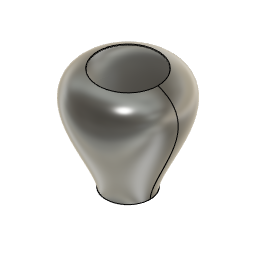
Vase_Homework (Autodesk Fusion 360 design; units mm, degrees)
Autodesk Fusion 360 part; units mm, degrees
sketch "Vase_Form" plane through (0, 0, 0) normal (0, 1, 0) x (1, 0, 0)
  spline S0 degree 5 poles (51.5187, 0) (51.5848, -1.6112) (51.9328, -5.0874) (53.1023, -11.0626) (55.9659, -20.5625) (61.704, -35.0058) (69.4537, -51.9393) (78.8368, -71.1094) (89.1317, -91.9905) (99.3864, -113.8767) (108.5272, -135.9665) (115.4599, -157.4412) (119.1828, -177.5466) (118.8878, -195.6666) (114.1203, -211.4335) (104.7239, -224.693) (93.5064, -233.2688) (83.0443, -238.5707) (75.1654, -241.6067) (71, -243) knots 0 0 0 0 0 0 0.066667 0.133333 0.2 0.266667 0.333333 0.4 0.466667 0.533333 0.6 0.666667 0.733333 0.8 0.866667 0.933333 1 1 1 1 1 1
  spline S1 degree 3 poles (53.0174, 0.0615) (53.2384, -5.3236) (55.0217, -12.7462) (58.4146, -22.0874) (61.2187, -29.8075) (65.129, -38.8618) (69.9141, -49.0892) (74.7583, -59.4428) (80.504, -71.0046) (86.4594, -83.2675) (94.4824, -99.7881) (102.8561, -117.5556) (109.2126, -134.8292) (114.0806, -148.0578) (117.7392, -160.9765) (119.248, -172.9258) (120.6759, -184.2343) (120.1641, -194.6786) (117.2946, -203.9293) (114.1604, -214.0334) (108.219, -222.6945) (99.5527, -229.7433) (92.1398, -235.7726) (82.7612, -240.6476) (71.4758, -244.4225) knots 0 0 0 0 0.140334 0.140334 0.140334 0.256315 0.256315 0.256315 0.373727 0.373727 0.373727 0.531903 0.531903 0.531903 0.653038 0.653038 0.653038 0.767678 0.767678 0.767678 0.892894 0.892894 0.892894 1 1 1 1
  spline S2 degree 5 poles (71, -243) (70.9155, -243.0511) (70.7546, -243.1512) (70.5382, -243.2955) (70.2999, -243.4758) (70.0918, -243.6796) (69.9811, -243.8599) (69.9755, -244.0149) (70.0789, -244.1437) (70.2865, -244.2475) (70.5901, -244.3282) (70.9034, -244.3758) (71.1754, -244.4026) (71.373, -244.4165) (71.4758, -244.4225) knots 0 0 0 0 0 0 0.1 0.2 0.3 0.4 0.5 0.6 0.7 0.8 0.9 1 1 1 1 1 1
  spline S3 degree 5 poles (53.0174, 0.0615) (53.0993, 0.2243) (53.1298, 0.5332) (52.7755, 0.946) (51.4902, 1.3939) (48.5075, 1.7803) (44.2426, 2.0049) (38.8498, 2.0873) (32.4979, 2.0487) (25.343, 1.9088) (17.5115, 1.6836) (10.7755, 1.444) (5.4807, 1.2337) (1.8446, 1.0801) (0, 1) knots 0 0 0 0 0 0 0.1 0.2 0.3 0.4 0.5 0.6 0.7 0.8 0.9 1 1 1 1 1 1
  line L0 (0, 1) -> (0, 0)
  line L1 (0, 0) -> (51.5187, 0)
  point P0 (69.9215, -52.6279)
  point P1 (118.5032, -182.876)
  point P2 (70, -244)
  point P3 (51.0124, 1.3778)
  dimension "d1" = -1.5
  constraint coincident L0.end L1.start
  constraint vertical L0
  constraint perpendicular L0 L1
revolve "Revolve1" add sketch "Vase_Form" angle 360 about axis through (0, 0, 1.75) along (0, 0, 1) contours 
named bodies: "Vase"
